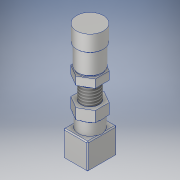
# Autodesk Inventor part: NeedleValveCAD
Saved by Autodesk Inventor 2017.3 (Build 213256000, 256)
## iProperties
Created: 2019-11-14
Part Number: NeedleValveCAD
Material: Generic
Document SubType Name: Modeling
Designer: guberti
Density: 1 g/cm^3
Appearance: Aluminum - Flat
Author: guberti
Autodesk Inventor part; units mm, degrees
ref_plane "YZ Plane" through (0, 0, 0) normal (1, 0, 0) x (0, 1, 0)
ref_plane "XZ Plane" through (0, 0, 0) normal (0, 1, 0) x (-1, 0, 0)
ref_plane "XY Plane" through (0, 0, 0) normal (0, 0, 1) x (1, 0, 0)
sketch "Sketch1" plane through (0, 0, 0) normal (0, 1, 0) x (-1, 0, 0)
  line L0 (-9.525, 11.43) -> (9.525, 11.43)
  line L1 (9.525, 11.43) -> (9.525, -11.43)
  line L2 (9.525, -11.43) -> (-9.525, -11.43)
  line L3 (-9.525, -11.43) -> (-9.525, 11.43)
  line L4 (-9.525, 11.43) -> (9.525, -11.43) construction
  line L5 (9.525, 11.43) -> (-9.525, -11.43) construction
  point P0 (0, 0)
  dimension "d0" = 19.05
  dimension "d1" = 22.86
  constraints: 12 end point, 2 midpoint, 2 parallel, 1 horizontal, 1 perpendicular
  measures "d0" distance of L1.end L2.end
  measures "d1" distance of L0.end L1.end
extrude "Extrusion1" add sketch "Sketch1" along normal blind 20.32
sketch "Sketch2" plane through (0, 20.32, 0) normal (0, 1, 0) x (1, 0, 0)
  circle A0 centre (0, 0) radius 9.144
  dimension "d4" = 18.288
  constraints: 1 centre point, 1 coincident
  measures "d4" diameter of A0
extrude "Extrusion2" add sketch "Sketch2" along normal blind 10.16
sketch "Sketch3" plane through (0, 30.48, 0) normal (0, 1, 0) x (1, 0, 0)
  line L0 (-9.525, 11.43) -> (-9.525, -11.43) projected
  line L1 (-9.525, 5.4993) -> (0, 10.9985)
  line L2 (0, 10.9985) -> (9.525, 5.4993)
  line L3 (9.525, 5.4993) -> (9.525, -5.4993)
  line L4 (9.525, -5.4993) -> (0, -10.9985)
  line L5 (0, -10.9985) -> (-9.525, -5.4993)
  line L6 (-9.525, -5.4993) -> (-9.525, 5.4993)
  point P0 (0, 0)
  point P1 (0, 0)
  point P2 (-9.525, 0)
  constraints: 12 end point, 2 midpoint, 1 coincident, 13 other
extrude "Extrusion3" add sketch "Sketch3" along normal blind 8.255
chamfer "Chamfer1" distance 0.7937 angle 45 13 edges at (9.525, 10.16, 11.43) (-9.525, 10.16, 11.43) (9.525, 10.16, -11.43) (-9.525, 10.16, -11.43) (0, 0, -11.43) (9.525, 0, 0) (0, 0, 11.43) (-9.525, 0, 0) (9.525, 20.32, 0) (0, 20.32, 11.43) (-9.525, 20.32, 0) (0, 20.32, -11.43) (-9.144, 30.48, 0)
sketch "Sketch4" plane through (0, 38.735, 0) normal (0, 1, 0) x (1, 0, 0)
  circle A0 centre (0, 0) radius 7.0485
  dimension "d12" = 14.097
  constraints: 1 centre point, 1 coincident
  measures "d12" diameter of A0
extrude "Extrusion4" add sketch "Sketch4" along normal blind 13.5128
sketch "Sketch5" plane through (0, 52.2478, 0) normal (0, 1, 0) x (1, 0, 0)
  circle A0 centre (0, 0) radius 8.255
  dimension "d15" = 16.51
  constraints: 1 centre point, 1 coincident
  measures "d15" diameter of A0
extrude "Extrusion5" add sketch "Sketch5" along normal blind 1.524
sketch "Sketch6" plane through (0, 53.7718, 0) normal (0, 1, 0) x (1, 0, 0)
  line L0 (0, -10.9985) -> (9.525, -5.4993) projected
  line L1 (0, -10.9985) -> (-9.525, -5.4993)
  line L2 (-9.525, -5.4993) -> (-9.525, 5.4993)
  line L3 (-9.525, 5.4993) -> (0, 10.9985)
  line L4 (0, 10.9985) -> (9.525, 5.4993)
  line L5 (9.525, 5.4993) -> (9.525, -5.4993)
  line L6 (9.525, -5.4993) -> (0, -10.9985)
  point P0 (0, 0)
  point P1 (0, 0)
  constraints: 12 end point, 1 coincident, 13 other
extrude "Extrusion6" add sketch "Sketch6" along normal blind 6.35
sketch "Sketch7" plane through (0, 60.1218, 0) normal (0, 1, 0) x (1, 0, 0)
  circle A0 centre (0, 0) radius 8.255
  dimension "d20" = 16.51
  constraints: 1 centre point, 1 coincident
  measures "d20" diameter of A0
extrude "Extrusion7" add sketch "Sketch7" along normal blind 1.524
sketch "Sketch8" plane through (0, 61.6458, 0) normal (0, 1, 0) x (1, 0, 0)
  circle A0 centre (0, 0) radius 9.525
  dimension "d23" = 19.05
  constraints: 1 centre point, 1 coincident
  measures "d23" diameter of A0
extrude "Extrusion8" add sketch "Sketch8" along normal blind 16.002
sketch "Sketch9" plane through (0, 77.6478, 0) normal (0, 1, 0) x (1, 0, 0)
  circle A0 centre (0, 0) radius 10.4775
  dimension "d26" = 20.955
  constraints: 1 centre point, 1 coincident
  measures "d26" diameter of A0
extrude "Extrusion9" add sketch "Sketch9" along normal blind 12.7
thread "Thread1" size "9/16-12 UNC" class "2A" standard "ANSI Unified Screw Threads" full length
chamfer "Chamfer2" distance 0.3969 angle 45 4 edges at (-8.255, 52.2478, 0) (-8.255, 53.7718, 0) (-8.255, 60.1218, 0) (-8.255, 61.6458, 0)
chamfer "Chamfer3" distance 0.3969 angle 45 1 edges at (-10.4775, 77.6478, 0)
body "Solid1"
